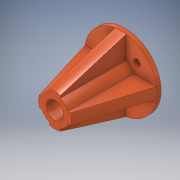
# Autodesk Inventor part: PieddeMat
Saved by Autodesk Inventor 2019 (Build 230136000, 136)
## iProperties
Created: 2019-07-30
Part Number: PieddeMat
Material: Plastique ABS
Document SubType Name: Modeling
Designer: Sébastien DI MERCURIO
Mass: 29.0117 g
Surface Area: 50.2812 cm^2
Volume: 27.3696 cm^3
Density: 1.06 g/cm^3
Appearance: Lisse - Orange clair
Author: Sébastien DI MERCURIO
Autodesk Inventor part; units mm, degrees
ref_plane "YZ Plane" through (0, 0, 0) normal (1, 0, 0) x (0, 1, 0)
ref_plane "XZ Plane" through (0, 0, 0) normal (0, 1, 0) x (-1, 0, 0)
ref_plane "XY Plane" through (0, 0, 0) normal (0, 0, 1) x (1, 0, 0)
sketch "Esquisse1" plane through (0, 0, 0) normal (0, 0, 1) x (1, 0, 0)
  circle A0 centre (0, 0) radius 16.5
  dimension "d0" = 33
  constraints: 1 centre point, 1 coincident
  measures "d0" diameter of A0
extrude "Extrusion1" add sketch "Esquisse1" along normal blind 32
sketch "Esquisse2" plane through (0, 0, 32) normal (0, 0, 1) x (1, 0, 0)
  circle A0 centre (0, 0) radius 4
  dimension "d3" = 8
  constraints: 1 centre point, 1 coincident
  measures "d3" diameter of A0
extrude "Extrusion2" cut sketch "Esquisse2" against normal through all
chamfer "Chanfrein1" distance 9 distance2 30 1 edges at (-16.5, 0, 32) measured on face at (12.1348, -1.6353, 32)
sketch "Esquisse3" plane through (0, 0, 32) normal (0, 0, 1) x (1, 0, 0)
  line L0 (2.5, 6) -> (2.5, 16.5)
  line L1 (6, 2.5) -> (16.5, 2.5)
  arc A0 (6, 2.5) -> (2.5, 6) centre (0, 0) ccw
  arc A1 (16.5, 2.5) -> (2.5, 16.5) centre (0, 0) ccw
  dimension "d9" = 2.5
  dimension "d10" = 2.5
  dimension "d11" = 6
  dimension "d12" = 16.5
  constraints: 5 end point, 4 point on circle, 2 centre point, 2 coincident, 1 horizontal, 1 vertical
  measures "d9" distance from line of point (0, 0) L0
  measures "d10" distance from line of point (0, 0) L1
  measures "d11" horizontal distance of point (0, 0) L1.start
  measures "d12" horizontal distance of point (0, 0) L1.end
extrude "Extrusion3" cut sketch "Esquisse3" against normal blind 30
pattern_circular "Réseau circulaire1" count 4 over 360 about axis through (0, 0, 32) along (0, 0, -1) of "Extrusion3"
sketch "Esquisse4" plane through (-16.3095, 2.5, 2) normal (0, 0, 1) x (1, 0, 0)
  circle A0 centre (8.8095, 5) radius 1.6
  point P0 (16.3095, -2.5)
  dimension "d18" = 3.2
  dimension "d19" = 7.5
  dimension "d20" = 7.5
  constraints: 1 centre point
  measures "d18" diameter of A0
  measures "d19" horizontal distance of point (16.31, -2.5) A0.centre
  measures "d20" horizontal distance of point (16.31, -2.5) A0.centre
extrude "Extrusion4" cut sketch "Esquisse4" against normal through all
pattern_circular "Réseau circulaire2" count 4 over 360 about axis through (0, 0, 32) along (0, 0, -1) of "Extrusion4"
equation "\"d10\" = d9"
equation "\"d20\" = d19"
